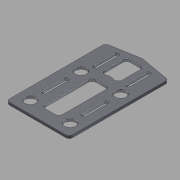
# Autodesk Inventor part: Camera Plate
Saved by Autodesk Inventor 2011 SP2 (Build 150309200, 309)
## iProperties
Created: 2015-02-19
Part Number: Camera Plate
Document SubType Name: Modeling
Designer: Greg Pavlik
Density: 1 g/cm^3
Author: Greg Pavlik
Autodesk Inventor part; units mm, degrees
ref_plane "YZ Plane" through (0, 0, 0) normal (1, 0, 0) x (0, 1, 0)
ref_plane "XZ Plane" through (0, 0, 0) normal (0, 1, 0) x (-1, 0, 0)
ref_plane "XY Plane" through (0, 0, 0) normal (0, 0, 1) x (1, 0, 0)
sketch "Sketch1" plane through (0, 0, 0) normal (0, 0, 1) x (1, 0, 0)
  line L0 (17.5, 53.2361) -> (17.5, 2)
  line L1 (15.5, 0) -> (-15.5, 0)
  line L2 (-17.5, 2) -> (-17.5, 53.2361)
  line L3 (0, 0) -> (0, 58) construction
  line L4 (0, 58) -> (-15.8473, 55.2057)
  line L5 (0, 58) -> (15.8473, 55.2057)
  arc A0 (15.5, 0) -> (17.5, 2) centre (15.5, 2) ccw
  arc A1 (-17.5, 2) -> (-15.5, 0) centre (-15.5, 2) ccw
  arc A2 (-15.8473, 55.2057) -> (-17.5, 53.2361) centre (-15.5, 53.2361) ccw
  arc A3 (17.5, 53.2361) -> (15.8473, 55.2057) centre (15.5, 53.2361) ccw
  circle A4 centre (-11, 7) radius 3
  circle A5 centre (11, 7) radius 3
  circle A6 centre (11, 35) radius 3
  circle A7 centre (-11, 35) radius 3
  line L6 (-2.75, 35) -> (2.75, 35)
  line L7 (4.75, 33) -> (4.75, 9)
  line L8 (2.75, 7) -> (-2.75, 7)
  line L9 (-4.75, 9) -> (-4.75, 33)
  line L10 (-2.75, 54) -> (2.75, 54)
  line L11 (4.75, 52) -> (4.75, 41.9776)
  line L12 (-4.75, 41.9776) -> (-4.75, 52)
  line L13 (12, 27) -> (12, 14.5)
  line L14 (10, 14.5) -> (10, 27)
  line L15 (-10, 27) -> (-10, 14.5)
  line L16 (-12, 14.5) -> (-12, 27)
  line L17 (-8, 53) -> (-8, 41)
  line L18 (-10, 41) -> (-10, 53)
  line L19 (10, 53) -> (10, 41)
  line L20 (8, 41) -> (8, 53)
  arc A8 (-10, 41) -> (-8, 41) centre (-9, 41) ccw
  arc A9 (8, 41) -> (10, 41) centre (9, 41) ccw
  arc A10 (10, 53) -> (8, 53) centre (9, 53) ccw
  arc A11 (-8, 53) -> (-10, 53) centre (-9, 53) ccw
  arc A12 (2.0167, 40.1169) -> (-2.0167, 40.1169) centre (0, 35) ccw
  arc A13 (-4.75, 41.9776) -> (-2.0167, 40.1169) centre (-2.75, 41.9776) ccw
  arc A14 (2.0167, 40.1169) -> (4.75, 41.9776) centre (2.75, 41.9776) ccw
  arc A15 (4.75, 52) -> (2.75, 54) centre (2.75, 52) ccw
  arc A16 (-2.75, 54) -> (-4.75, 52) centre (-2.75, 52) ccw
  arc A17 (-12, 14.5) -> (-10, 14.5) centre (-11, 14.5) ccw
  arc A18 (-10, 27) -> (-12, 27) centre (-11, 27) ccw
  arc A19 (12, 27) -> (10, 27) centre (11, 27) ccw
  arc A20 (10, 14.5) -> (12, 14.5) centre (11, 14.5) ccw
  arc A21 (-2.75, 35) -> (-4.75, 33) centre (-2.75, 33) ccw
  arc A22 (4.75, 33) -> (2.75, 35) centre (2.75, 33) ccw
  arc A23 (2.75, 7) -> (4.75, 9) centre (2.75, 9) ccw
  arc A24 (-4.75, 9) -> (-2.75, 7) centre (-2.75, 9) ccw
  line L21 (-11, 35) -> (-11, 7) construction
  point P0 (-4.75, 37.7726)
  point P1 (4.75, 37.7726)
  dimension "d0" = 35
  dimension "d1" = 160
  dimension "d2" = 58
  dimension "d3" = 2
  dimension "d4" = 2
  dimension "d5" = 2
  dimension "d7" = 7
  dimension "d8" = 6
  dimension "d9" = 35
  dimension "d10" = 6.5
  dimension "d11" = 14.5
  dimension "d12" = 12.5
  dimension "d13" = 1
  dimension "d14" = 7
  dimension "d15" = 28
  dimension "d16" = 12.75
  dimension "d17" = 41
  dimension "d18" = 18
  dimension "d19" = 53
  dimension "d20" = 54
  dimension "d21" = 9.5
  dimension "d22" = 19
  dimension "d23" = 5.5
  dimension "d32" = 22
  constraints: 45 point on circle, 44 end point, 39 tangent, 25 centre point, 11 equal radius, 11 parallel, 4 point on line, 3 perpendicular, 2 coincident, 2 horizontal, 1 midpoint, 1 vertical, 18 other
  measures "d0" distance between parallel lines of L0 L2
  measures "d1" angle of L5 L4
  measures "d2" distance from line of L1 L3.end
  measures "d3" radius of A0
  measures "d4" radius of A13
  measures "d5" radius of A21
  measures "d7" distance from line of A4.centre L1
  measures "d8" diameter of A5
  measures "d9" distance from line of L1 A7.centre
  measures "d10" distance from line of A17.centre L2
  measures "d11" distance from line of L1 A17.centre
  measures "d12" distance of A18.centre A17.centre
  measures "d13" radius of A19
  measures "d14" distance between parallel lines of L1 L8
  measures "d15" distance between parallel lines of L6 L8
  measures "d16" distance between parallel lines of L0 L7
  measures "d17" distance from line of L1 A8.centre
  measures "d18" distance of A10.centre A11.centre
  measures "d19" distance from line of L1 A11.centre
  measures "d20" distance between parallel lines of L1 L10
  measures "d21" distance between parallel lines of L11 L12
  measures "d22" distance from line of A12.centre L10
  measures "d23" radius of A12
  measures "d32" distance from line of A5.centre L21
extrude "Extrusion1" add sketch "Sketch1" along normal mid plane 1.5
chamfer "Chamfer1" distance 0.15 angle 45 72 edges at (-4.75, 21, 0.75) (-4.1642, 34.4142, 0.75) (0, 35, 0.75) (4.1642, 34.4142, 0.75) (4.75, 21, 0.75) (4.1642, 7.5858, 0.75) (0, 7, 0.75) (-4.1642, 7.5858, 0.75) (-4.75, 21, -0.75) (-4.1642, 7.5858, -0.75) (0, 7, -0.75) (4.1642, 7.5858, -0.75) (4.75, 21, -0.75) (4.1642, 34.4142, -0.75) (0, 35, -0.75) (-4.1642, 34.4142, -0.75) (-4.75, 46.9888, 0.75) (-4.1642, 53.4142, 0.75) (0, 54, 0.75) (4.1642, 53.4142, 0.75) (4.75, 46.9888, 0.75) (3.8755, 40.3244, 0.75) (0, 40.5, 0.75) (-3.8755, 40.3244, 0.75) (-4.75, 46.9888, -0.75) (-3.8755, 40.3244, -0.75) (0, 40.5, -0.75) (3.8755, 40.3244, -0.75) (4.75, 46.9888, -0.75) (4.1642, 53.4142, -0.75) (0, 54, -0.75) (-4.1642, 53.4142, -0.75) (-8, 47, 0.75) (-9, 40, 0.75) (-10, 47, 0.75) (-9, 54, 0.75) (-8, 47, -0.75) (-9, 54, -0.75) (-10, 47, -0.75) (-9, 40, -0.75) (8, 47, 0.75) (9, 54, 0.75) (10, 47, 0.75) (9, 40, 0.75) (10, 47, -0.75) (9, 54, -0.75) (8, 47, -0.75) (9, 40, -0.75) (8, 35, 0.75) (11, 28, -0.75) (10, 20.75, -0.75) (11, 13.5, -0.75) (12, 20.75, -0.75) (8, 7, -0.75) (10, 20.75, 0.75) (11, 28, 0.75) (12, 20.75, 0.75) (11, 13.5, 0.75) (-12, 20.75, 0.75) (-11, 28, 0.75) (-10, 20.75, 0.75) (-11, 13.5, 0.75) (-12, 20.75, -0.75) (-11, 13.5, -0.75) (-10, 20.75, -0.75) (-11, 28, -0.75) (8, 35, -0.75) (8, 7, 0.75) (-14, 7, 0.75) (-14, 35, 0.75) (-14, 35, -0.75) (-14, 7, -0.75)
chamfer "Chamfer2" distance 0.15 angle 45 18 edges at (17.0321, 54.5217, -0.75) (7.9236, 56.6028, -0.75) (17.5, 27.618, -0.75) (16.9142, 0.5858, -0.75) (0, 0, -0.75) (-16.9142, 0.5858, -0.75) (-17.5, 27.618, -0.75) (-17.0321, 54.5217, -0.75) (-7.9236, 56.6028, -0.75) (17.0321, 54.5217, 0.75) (17.5, 27.618, 0.75) (16.9142, 0.5858, 0.75) (0, 0, 0.75) (-16.9142, 0.5858, 0.75) (-17.5, 27.618, 0.75) (-17.0321, 54.5217, 0.75) (-7.9236, 56.6028, 0.75) (7.9236, 56.6028, 0.75)
body "Solid1"
